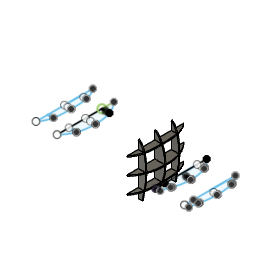
Shelf (Autodesk Fusion 360 design; units mm, degrees)
Autodesk Fusion 360 part; units mm, degrees
note: some values were not read from the file. Set by a fixed rule: which sketch regions a step uses.
sketch "Sketch1" plane through (0, 0, 0) normal (0, 0, 1) x (1, 0, 0) in component "Component"
  line L0 (0, 0) -> (0, 709)
  line L1 (0, 354.5) -> (140, 354.5) construction
  line L2 (0, 354.5) -> (0, 575.9)
  line L3 (0, 124.5) -> (94.6571, 124.5) construction
  line L4 (60, 0) -> (0, 0)
  line L5 (400.6534, 354.5) -> (400.6534, 584.5)
  line L6 (400.6534, 354.5) -> (505.0275, 354.5) construction
  line L7 (400.6534, 124.5) -> (477.548, 124.5) construction
  line L8 (400.6534, 0) -> (400.6534, 709)
  line L9 (460, 0) -> (400.6534, 0)
  line L10 (400.6534, 584.5) -> (478.2014, 584.5) construction
  line L11 (-1337.528, 585.6533) -> (-1233.154, 585.6533) construction
  line L12 (-1337.8811, 355.6536) -> (-1197.8811, 355.6536) construction
  line L13 (0, 584.5) -> (94.6571, 584.5) construction
  line L14 (-1643.807, 376.7828) -> (-1643.807, 589.5796)
  line L15 (-1643.807, 368.1796) -> (-1549.15, 368.1796) construction
  line L16 (-1643.807, 598.1796) -> (-1566.259, 598.1796) construction
  spline S0 degree 5 poles (-1549.15, 368.1796) (-1549.15, 376.6058) (-1549.2112, 393.6073) (-1549.4863, 419.5568) (-1550.2981, 454.9209) (-1552.5188, 499.6662) (-1556.5685, 544.0061) (-1563.0982, 586.9778) (-1572.6615, 627.771) (-1585.4861, 665.996) (-1601.555, 701.5954) (-1616.9305, 728.039) (-1629.8378, 746.7781) (-1639.0495, 758.7922) (-1643.807, 764.6796) knots 0 0 0 0 0 0 0.1 0.2 0.3 0.4 0.5 0.6 0.7 0.8 0.9 1 1 1 1 1 1
  line L17 (-1549.15, 326.3333) -> (-1549.15, 410.0259)
  spline S1 degree 5 poles (-1549.15, 368.1796) (-1549.15, 359.7534) (-1549.2112, 342.752) (-1549.4863, 316.8024) (-1550.2981, 281.4383) (-1552.5188, 236.693) (-1556.5685, 192.3532) (-1563.0982, 149.3814) (-1572.6615, 108.5883) (-1585.4861, 70.3632) (-1601.555, 34.7638) (-1616.9305, 8.3202) (-1629.8378, -10.4189) (-1639.0495, -22.433) (-1643.807, -28.3204) knots 0 0 0 0 0 0 0.1 0.2 0.3 0.4 0.5 0.6 0.7 0.8 0.9 1 1 1 1 1 1
  line L18 (-1617.6653, 732.3293) -> (-1669.9487, 797.03)
  line L19 (-1549.15, 410.0259) -> (-1549.15, 326.3333)
  line L20 (-1617.6653, 4.03) -> (-1669.9487, -60.6707)
  line L21 (-1337.528, 125.6539) -> (-1233.154, 125.6539) construction
  spline S2 degree 5 poles (-1197.8811, 355.6536) (-1197.8241, 365.3466) (-1197.9658, 384.579) (-1198.9449, 412.9662) (-1201.7966, 449.8811) (-1208.0512, 494.376) (-1217.1771, 537.0842) (-1229.3761, 577.8584) (-1244.8026, 616.5901) (-1263.4135, 653.3122) (-1285.0533, 688.1408) (-1304.6634, 714.5853) (-1320.6155, 733.6601) (-1331.7991, 746.0434) (-1337.528, 752.1518) knots 0 0 0 0 0 0 0.1 0.2 0.3 0.4 0.5 0.6 0.7 0.8 0.9 1 1 1 1 1 1
  spline S3 degree 5 poles (-1197.8811, 355.6536) (-1197.8241, 345.9605) (-1197.9658, 326.7282) (-1198.9449, 298.341) (-1201.7966, 261.4261) (-1208.0512, 216.9312) (-1217.1771, 174.223) (-1229.3761, 133.4488) (-1244.8026, 94.7171) (-1263.4135, 57.995) (-1285.0533, 23.1664) (-1304.6634, -3.2781) (-1320.6155, -22.3529) (-1331.7991, -34.7362) (-1337.528, -40.8446) knots 0 0 0 0 0 0 0.1 0.2 0.3 0.4 0.5 0.6 0.7 0.8 0.9 1 1 1 1 1 1
  line L22 (-1198.1716, 306.1963) -> (-1197.5906, 405.1109)
  line L23 (-1305.8031, 718.3259) -> (-1369.253, 785.9777)
  line L24 (-1198.1716, 405.1109) -> (-1197.5906, 306.1963)
  line L25 (-1305.8031, -7.0187) -> (-1369.253, -74.6705)
  line L26 (-1267.8811, 355.6536) -> (-1267.8811, 347.0536)
  line L27 (-1267.8811, 347.0536) -> (-1337.528, 347.0536)
  line L28 (-1267.8811, 355.6536) -> (-1267.8811, 364.2536)
  line L29 (-1267.8811, 364.2536) -> (-1337.528, 364.2536)
  line L30 (-1285.341, 585.6533) -> (-1285.341, 577.0533)
  line L31 (-1285.341, 577.0533) -> (-1337.528, 577.0533)
  line L32 (-1285.341, 585.6533) -> (-1285.341, 594.2533)
  line L33 (-1285.341, 594.2533) -> (-1337.528, 594.2533)
  line L34 (-1337.528, 364.2536) -> (-1337.528, 577.0533)
  line L35 (-1337.528, 594.2533) -> (-1337.528, 752.1518)
  line L36 (-1285.341, 134.2539) -> (-1337.528, 134.2539)
  line L37 (-1285.341, 125.6539) -> (-1285.341, 134.2539)
  line L38 (-1285.341, 125.6539) -> (-1285.341, 117.0539)
  line L39 (-1285.341, 117.0539) -> (-1337.528, 117.0539)
  line L40 (-1337.528, -40.8482) -> (-1337.528, 117.0539)
  line L41 (-1337.528, 134.2539) -> (-1337.528, 347.0536)
  line L42 (-1605.033, 598.1796) -> (-1605.033, 606.7796)
  line L43 (-1605.033, 606.7796) -> (-1643.807, 606.7796)
  line L44 (-1605.033, 589.5796) -> (-1643.807, 589.5796)
  line L45 (-1605.033, 598.1796) -> (-1605.033, 589.5796)
  line L46 (-1643.807, 606.7796) -> (-1643.807, 764.6796)
  line L47 (-1596.4785, 368.1796) -> (-1596.4785, 376.7796)
  line L48 (-1596.4785, 376.7796) -> (-1643.807, 376.7828)
  line L49 (-1596.4785, 368.1796) -> (-1596.4785, 359.5796)
  line L50 (-1596.4785, 359.5796) -> (-1643.807, 359.5765)
  line L51 (-1643.807, 376.7828) -> (-1643.807, 589.5796)
  line L52 (-1643.807, 606.7796) -> (-1643.807, 589.5796) construction
  line L53 (-1605.033, 146.7796) -> (-1643.807, 146.7796)
  line L54 (-1605.033, 138.1796) -> (-1605.033, 146.7796)
  line L55 (-1605.033, 129.5796) -> (-1643.807, 129.5796)
  line L56 (-1605.033, 138.1796) -> (-1605.033, 129.5796)
  line L57 (-1643.807, -28.3204) -> (-1643.807, 129.5796)
  line L58 (-1643.807, 146.7796) -> (-1643.807, 359.5765)
  line L59 (70, 354.5) -> (70, 363.1)
  line L60 (70, 354.5) -> (70, 345.9)
  line L61 (47.3285, 584.5) -> (47.3285, 593.1)
  line L62 (47.3285, 584.5) -> (47.3285, 575.9)
  line L63 (47.3285, 124.5) -> (47.3285, 133.1)
  line L64 (47.3285, 124.5) -> (47.3285, 115.9)
  line L65 (452.8405, 354.5) -> (452.8405, 363.1)
  line L66 (452.8405, 354.5) -> (452.8405, 345.9)
  line L67 (438.76, 584.5356) -> (438.7596, 593.1356)
  line L68 (438.76, 584.5356) -> (438.7606, 575.952)
  line L69 (438.774, 124.5) -> (438.774, 133.1)
  line L70 (438.774, 124.5) -> (438.774, 115.9)
  line L71 (47.3285, 593.1) -> (90.6994, 593.1)
  line L72 (47.3285, 575.9) -> (98.3999, 575.9)
  line L73 (70, 363.1) -> (139.9509, 363.1)
  line L74 (70, 345.9) -> (139.9449, 345.9)
  line L75 (47.3285, 133.1) -> (98.3802, 133.1)
  line L76 (47.3285, 115.9) -> (90.924, 115.9)
  line L77 (438.774, 133.1) -> (479.9553, 133.1)
  spline S4 degree 5 poles (90.6994, 593.1) (89.2283, 596.209) (81.2165, 612.7189) (65.584, 640.9011) (48.0847, 665.7514) (28.7547, 686.763) (9.8458, 702.1636) (0, 709) knots 0.554213 0.554213 0.554213 0.554213 0.554213 0.554213 0.6 0.8 1 1 1 1 1 1
  line L78 (98.3825, 576.8627) -> (83.0163, 609.3373)
  line L79 (11.6564, 700.9064) -> (-11.6564, 717.0936)
  spline S5 degree 5 poles (139.9509, 363.1) (139.7301, 382.3414) (137.9721, 421.1557) (132.3196, 466.9254) (122.8436, 508.4908) (110.3653, 546.3144) (101.5473, 568.4621) (98.3999, 575.9) knots 0.01632 0.01632 0.01632 0.01632 0.01632 0.01632 0.2 0.4 0.5047 0.5047 0.5047 0.5047 0.5047 0.5047
  line L80 (140.254, 336.6922) -> (139.6479, 389.5078)
  line L81 (105.9592, 558.0361) -> (90.8405, 593.7639)
  spline S6 degree 5 poles (90.924, 115.9) (89.4266, 112.3406) (85.8459, 103.5381) (80.6515, 89.6012) (74.5511, 70.7164) (68.2523, 47.2018) (64.0892, 27.7294) (61.7231, 13.6364) (60.5131, 4.502) (60, 0) knots 0.065011 0.065011 0.065011 0.065011 0.065011 0.065011 0.2 0.4 0.6 0.8 1 1 1 1 1 1
  line L82 (96.2825, 128.638) -> (85.5655, 103.162)
  line L83 (61.2385, 10.8664) -> (58.7615, -10.8664)
  spline S7 degree 5 poles (139.9449, 345.9) (139.8243, 336.5369) (139.2011, 316.482) (137.0478, 286.8211) (131.9333, 249.0909) (123.0436, 206.9091) (113.9266, 174.7511) (106.1954, 152.5019) (100.8079, 138.8973) (98.3802, 133.1) knots 0.030861 0.030861 0.030861 0.030861 0.030861 0.030861 0.2 0.4 0.6 0.8 0.953806 0.953806 0.953806 0.953806 0.953806 0.953806
  line L84 (140.2844, 372.2447) -> (139.6054, 319.5553)
  line L85 (105.8752, 150.9978) -> (90.8852, 115.2022)
  line L86 (438.774, 115.9) -> (475.1869, 115.9)
  spline S8 degree 5 poles (475.1869, 115.9) (474.238, 112.2307) (472.063, 103.2249) (469.225, 89.04) (466.5009, 69.9403) (464.2659, 46.3502) (462.7184, 27.0461) (461.4415, 13.229) (460.4962, 4.3536) (460, 0) knots 0.063628 0.063628 0.063628 0.063628 0.063628 0.063628 0.2 0.4 0.6 0.8 1 1 1 1 1 1
  line L87 (478.5171, 128.7784) -> (471.8567, 103.0216)
  line L88 (461.1919, 10.4572) -> (458.8081, -10.4572)
  line L89 (452.8405, 363.1) -> (505.005, 363.1)
  line L90 (452.8405, 345.9) -> (504.9906, 345.9)
  spline S9 degree 5 poles (504.9906, 345.9) (504.9184, 336.8623) (504.5676, 317.3756) (503.384, 288.2996) (500.5685, 250.8684) (495.5022, 208.4527) (490.0015, 175.7944) (485.0958, 153.0601) (481.5699, 139.0894) (479.9553, 133.1) knots 0.031824 0.031824 0.031824 0.031824 0.031824 0.031824 0.2 0.4 0.6 0.8 0.955003 0.955003 0.955003 0.955003 0.955003 0.955003
  line L91 (505.1939, 371.3164) -> (504.7874, 320.4836)
  line L92 (484.8705, 151.3323) -> (475.04, 114.8677)
  line L93 (438.7596, 593.1356) -> (475.5996, 593.1374)
  line L94 (438.7606, 575.952) -> (480.6063, 575.9548)
  spline S10 degree 5 poles (505.005, 363.1) (504.8974, 381.4546) (504.0059, 418.8119) (501.0592, 464.2441) (495.9075, 506.2377) (488.4797, 544.9127) (482.7871, 567.8898) (480.6063, 575.9548) knots 0.017056 0.017056 0.017056 0.017056 0.017056 0.017056 0.2 0.4 0.512081 0.512081 0.512081 0.512081 0.512081 0.512081
  line L95 (505.1542, 337.6508) -> (504.8558, 388.5492)
  line L96 (485.5287, 557.751) -> (475.6839, 594.1587)
  spline S11 degree 5 poles (475.5996, 593.1374) (474.752, 595.8394) (469.468, 612.1938) (458.5304, 640.5688) (445.0745, 665.6454) (428.4916, 686.7376) (410.4267, 702.2039) (400.6534, 709) knots 0.560836 0.560836 0.560836 0.560836 0.560836 0.560836 0.6 0.8 1 1 1 1 1 1
  line L97 (480.7462, 576.7303) -> (470.453, 609.5445)
  line L98 (412.0593, 701.0686) -> (389.2476, 716.9314)
  point P0 (0, 124.5)
  point P1 (400.6534, 124.5)
  point P2 (-1566.259, 138.1796)
  point P3 (-1233.154, 125.6539)
  dimension "d1" = 709
  dimension "d2" = 140
  dimension "d3" = 230
  dimension "d7" = 709
  dimension "d9" = 230
  dimension "d10" = 77.548
  dimension "d11" = 793
  dimension "d12" = 230
  dimension "d14" = 94.6571
  dimension "d24" = 94.657
  dimension "d25" = 230
  dimension "d26" = 77.548
  dimension "d53" = 793
  dimension "d55" = 140
  dimension "d59" = 8.6
  dimension "d60" = 8.6
  dimension "d61" = 52.187
  dimension "d63" = 104.374
  dimension "d64" = 8.6
  dimension "d65" = 52.187
  dimension "d66" = 8.6
  dimension "d67" = 8.6
  dimension "d68" = 8.6
  dimension "d69" = 8.6
  dimension "d70" = 8.6
  dimension "d71" = 8.6
  dimension "d72" = 8.6
  dimension "d73" = 8.6
  dimension "d74" = 8.6
  constraint coincident L0.start L4.end
  constraint vertical L0
  constraint midpoint L0 L1.start
  constraint perpendicular L0 L1
  constraint symmetric L0.end L1 L0.start
  constraint coincident L0 L13.start
  constraint symmetric L1 L13.start P0
  constraint coincident P0 L3.start
  constraint perpendicular L0 L3
  constraint perpendicular L0 L4
  constraint vertical L8
  constraint midpoint L5.start L8
  constraint perpendicular L6 L8
  constraint symmetric L8.start L8.end L6
  constraint coincident L5.end L8
  constraint symmetric L5.end P1 L6
  constraint coincident P1 L7.start
  constraint perpendicular L7 L8
  constraint perpendicular L8 L9
  constraint perpendicular L5 L10
  constraint vertical L40
  constraint perpendicular L12 L40
  constraint perpendicular L11 L40
  constraint perpendicular L0 L13
  constraint vertical L57
  constraint perpendicular L15 L57
  constraint perpendicular L14 L15
  constraint perpendicular L14 L16
  constraint midpoint L15.end L17
  constraint midpoint S0.end L18
  constraint symmetric L16.end L15 P2
  constraint symmetric S0.end L15 S1.end
  constraint symmetric S0.start L15 S1.start
  constraint symmetric L15 L17.start L17.end
  constraint symmetric L15 L17.end L17.start
  constraint symmetric L15 L18.start L20.start
  constraint symmetric L15 L18.end L20.end
  constraint symmetric L11.start L12 L21.start
  constraint symmetric L11.end L12 P3
  constraint midpoint L12.end L22
  constraint midpoint S2.end L23
  constraint symmetric S2.start L12 S3.start
  constraint symmetric S2.end L12 S3.end
  constraint symmetric L12 L22.start L24.start
  constraint symmetric L12 L22.end L24.end
  constraint symmetric L12 L23.start L25.start
  constraint symmetric L12 L23.end L25.end
  constraint midpoint L12 L26.start
  constraint perpendicular L12 L26
  constraint perpendicular L27 L40
  constraint symmetric L12 L26.start L28.start
  constraint symmetric L12 L26.end L28.end
  constraint symmetric L12 L27.end L29.end
  constraint collinear L34 L40
  constraint midpoint L11 L30.start
  constraint perpendicular L11 L30
  constraint perpendicular L31 L34
  constraint symmetric L11 L30.start L32.start
  constraint symmetric L11 L30.end L32.end
  constraint symmetric L11 L31.end L33.end
  constraint collinear L34 L35
  constraint collinear L40 L41
  constraint midpoint L16 L42.start
  constraint perpendicular L16 L42
  constraint coincident L43.end L57
  constraint perpendicular L43 L57
  constraint symmetric L16 L42.start L45.start
  constraint symmetric L16 L42.end L44.start
  constraint symmetric L16 L43.end L14.end
  constraint collinear L46 L57
  constraint midpoint L15 L47.start
  constraint perpendicular L15 L47
  constraint symmetric L15 L47.start L49.start
  constraint symmetric L15 L47.end L49.end
  constraint symmetric L15 L14.start L50.end
  constraint collinear L51 L57
  constraint coincident L16.start L52
  constraint collinear L57 L58
  constraint equal L54 L56
  constraint equal L37 L38
  constraint coincident L54.start L56.start
  constraint coincident L37.start L38.start
  constraint coincident L21 L37.start
  constraint midpoint L1 L59.start
  constraint perpendicular L1 L59
  constraint symmetric L1 L59.start L60.start
  constraint symmetric L1 L59.end L60.end
  constraint midpoint L13 L61.start
  constraint perpendicular L13 L61
  constraint symmetric L13 L61.start L62.start
  constraint symmetric L13 L61.end L62.end
  constraint coincident L63.start L64.start
  constraint equal L63 L64
  constraint midpoint L6 L65.start
  constraint perpendicular L6 L65
  constraint symmetric L6 L65.start L66.start
  constraint symmetric L6 L65.end L66.end
  constraint coincident L67.start L68.start
  constraint coincident L69.start L70.start
  constraint perpendicular L61 L71
  constraint perpendicular L62 L72
  constraint perpendicular L59 L73
  constraint perpendicular L60 L74
  constraint perpendicular L63 L75
  constraint perpendicular L64 L76
  constraint midpoint L71.end L78
  constraint midpoint L0.end L79
  constraint midpoint L73.end L80
  constraint midpoint L72.end L81
  constraint midpoint L76.end L82
  constraint midpoint L4.start L83
  constraint midpoint L74.end L84
  constraint midpoint L75.end L85
  constraint midpoint L86.end L87
  constraint midpoint L9.start L88
  constraint midpoint L90.end L91
  constraint midpoint L77.end L92
  constraint perpendicular L67 L93
  constraint perpendicular L68 L94
  constraint midpoint L89.end L95
  constraint midpoint L94.end L96
  constraint midpoint L93.end L97
  constraint midpoint L8.end L98
  measures "d1" distance of L0.start L0.end
  measures "d2" distance of L1.start L1.end
  measures "d3" distance of L1.start L13.start
  measures "d7" distance of L8.end L8.start
  measures "d9" distance of L5.end L5.start
  measures "d10" distance of L5.end L10.end
  measures "d11" distance of L40.start S2.end
  measures "d12" distance of L12.start L11.start
  measures "d14" distance of L13.start L13.end
  measures "d24" distance of L15.start L15.end
  measures "d25" distance of L15.start L16.start
  measures "d26" distance of L16.end L16.start
  measures "d53" distance of S0.end S1.end
  measures "d55" distance of L12.start L12.end
  measures "d59" distance of L26.start L26.end
  measures "d60" distance of L30.start L30.end
  measures "d61" distance of L32.end L33.end
  measures "d63" distance of L11.start L11.end
  measures "d64" distance of L37.start L38.end
  measures "d65" distance of L36.start L36.end
  measures "d66" distance of L42.start L42.end
  measures "d67" distance of L47.start L47.end
  measures "d68" distance of L54.start L53.start
  measures "d69" distance of L59.start L59.end
  measures "d70" distance of L61.start L61.end
  measures "d71" distance of L63.start L63.end
  measures "d72" distance of L65.start L65.end
  measures "d73" distance of L67.start L67.end
  measures "d74" distance of L69.end L69.start
extrude "Extrude4" add sketch "Sketch1" along normal blind 15.2 contours L0 L2 L4 L59 L60 L61 L62 L63 L64 L71 L72 L73 L74 L75 L76 S4 S5 S6 S7 | L5 L8 L9 L65 L66 L67 L68 L69 L70 L77 L86 S8 L89 L90 S9 L93 L94 S10 S11 | L14 S0 S1 L42 L43 L44 L45 L46 L47 L48 L49 L50 L51 L53 L54 L55 L56 L57 L58 | S2 L24 | S3 L22 | S2 S3 L22 L24 L26 L27 L28 L29 L30 L31 L32 L33 L34 L35 L36 L37 L38 L39 L40 L41 makes body 1 at (-1293.298, 241.2726, 0) makes body 2 at (39.9441, 481.4364, 0) makes body 3 at (-1615.809, 226.6085, 0) makes body 4 at (433.7072, 468.424, 0) in component "Component"
move_body "Move11" bodies 2 to x (1, 0, 0) y (0, 0, 1) z (0, -1, 0) at (0, 0, 0) in component "Component"
move_body "Move12" bodies 4 to x (1, 0, 0) y (0, 0, 1) z (0, -1, 0) at (0, 0, 0) in component "Component"
move_body "Move13" bodies 4 to x (1, 0, 0) y (0, 1, 0) z (0, 0, 1) at (-400.6534, 0, 0) in component "Component"
move_body "Move14" bodies 4 to x (1, 0, 0) y (0, 1, 0) z (0, 0, 1) at (0, 230, 0) in component "Component"
copy_body "CopyPasteBodies3" bodies 4 makes body 5 in component "Component"
move_body "Move15" bodies 5 to x (1, 0, 0) y (0, 1, 0) z (0, 0, 1) at (0, -460, 0) in component "Component"
move_body "Move16" bodies 1 to x (1, 0, 0) y (0, 1, 0) z (0, 0, 1) at (1337.8811, -362.2536, 347.9) in component "Component"
move_body "Move17" bodies 3 to x (1, 0, 0) y (0, 1, 0) z (0, 0, 1) at (1643.807, -374.7796, 577.9) in component "Component"
copy_body "CopyPasteBodies4" bodies 3 makes body 6 in component "Component"
move_body "Move18" bodies 6 to x (1, 0, 0) y (0, 1, 0) z (0, 0, 1) at (0, 0, -460) in component "Component"
extrude "Extrude1" [suppressed] in component "Component"
extrude "Extrude2" [suppressed] in component "Component"
extrude "Extrude3" [suppressed] in component "Component"
move_body "Move1" [suppressed] in component "Component"
move_body "Move2" [suppressed] in component "Component"
move_body "Move3" [suppressed] in component "Component"
move_body "Move4" [suppressed] in component "Component"
copy_body "CopyPasteBodies1" [suppressed] in component "Component"
move_body "Move5" [suppressed] in component "Component"
move_body "Move6" [suppressed] in component "Component"
move_body "Move7" [suppressed] in component "Component"
move_body "Move8" [suppressed] in component "Component"
move_body "Move9" [suppressed] in component "Component"
copy_body "CopyPasteBodies2" [suppressed] in component "Component"
move_body "Move10" [suppressed] in component "Component"
component "Component" placed x (1, 0, 0) y (0, 1, 0) z (0, 0, 1) at (0, 0, 0)
equation "d1 = Height"
equation "d2 = Depth_Belly_MiddlePoint"
equation "d3 = Height_Cell"
equation "d7 = Height"
equation "d9 = Height_Cell"
equation "d11 = Width"
equation "d12 = Height_Cell"
equation "d25 = Height_Cell"
equation "Height_Cell = 230 mm"
equation "Height = 709 mm"
equation "Width = 793 mm"
equation "d53 = Width"
equation "Depth_Belly_MiddlePoint = 140 mm"
equation "d55 = Depth_Belly_MiddlePoint"
equation "Depth_Side_MiddlePoint = 104.374 mm"
equation "MaterialThickness = 15.2 mm"
equation "Kerf = 2 mm"
equation "d59 = ( MaterialThickness + Kerf ) / 2"
equation "d60 = ( MaterialThickness + Kerf ) / 2"
equation "d63 = Depth_Side_MiddlePoint"
equation "d64 = ( MaterialThickness + Kerf ) / 2"
equation "d66 = ( MaterialThickness + Kerf ) / 2"
equation "d67 = ( MaterialThickness + Kerf ) / 2"
equation "d68 = ( MaterialThickness + Kerf ) / 2"
equation "d69 = ( MaterialThickness + Kerf ) / 2"
equation "d70 = ( MaterialThickness + Kerf ) / 2"
equation "d71 = ( MaterialThickness + Kerf ) / 2"
equation "d72 = ( MaterialThickness + Kerf ) / 2"
equation "d73 = ( MaterialThickness + Kerf ) / 2"
equation "d74 = ( MaterialThickness + Kerf ) / 2"
equation "d79 = Height"
equation "d80 = Depth_Belly_MiddlePoint"
equation "d81 = Height_Cell"
equation "d82 = Height"
equation "d83 = Height_Cell"
equation "d85 = Width"
equation "d86 = Height_Cell"
equation "d88 = Height_Cell"
equation "d90 = Width"
equation "d91 = Depth_Belly_MiddlePoint"
equation "d92 = ( MaterialThickness + Kerf ) / 2"
equation "d93 = ( MaterialThickness + Kerf ) / 2"
equation "d95 = Depth_Side_MiddlePoint"
equation "d96 = ( MaterialThickness + Kerf ) / 2"
equation "d98 = ( MaterialThickness + Kerf ) / 2"
equation "d99 = ( MaterialThickness + Kerf ) / 2"
equation "d100 = ( MaterialThickness + Kerf ) / 2"
equation "d101 = ( MaterialThickness + Kerf ) / 2"
equation "d102 = ( MaterialThickness + Kerf ) / 2"
equation "d103 = ( MaterialThickness + Kerf ) / 2"
equation "d104 = ( MaterialThickness + Kerf ) / 2"
equation "d105 = ( MaterialThickness + Kerf ) / 2"
equation "d106 = ( MaterialThickness + Kerf ) / 2"
